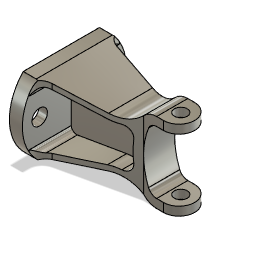
0.885.1264 - Pied de hauban - IGTE 21481_222676 (Autodesk Fusion 360 design; units mm, degrees)
Autodesk Fusion 360 part; units mm, degrees
sketch "Sketch1" plane through (0, 0, 0) normal (0, 0, 1) x (1, 0, 0)
  line L0 (0, 0) -> (0, 40)
  line L1 (0, 40) -> (15, 40)
  line L2 (0, 0) -> (0, -40)
  line L3 (0, -40) -> (15, -40)
  line L4 (15, 26.7964) -> (15, -26.7964)
  line L5 (15, 0) -> (85, 0) construction
  line L6 (85, 0) -> (85, 22) construction
  line L7 (85, 0) -> (85, -22) construction
  line L8 (79.9016, 28.874) -> (15, 40)
  line L9 (138, 0) -> (138, 68.5674) construction
  line L10 (113, 0) -> (113, 68.5674) construction
  line L11 (138, 46) -> (154, 46)
  line L12 (138, 36) -> (154, 36)
  line L13 (154, 46) -> (154, 36)
  line L14 (138, -36) -> (128.0077, -36)
  line L15 (138, -46) -> (154, -46)
  line L16 (138, -36) -> (154, -36)
  line L17 (154, -46) -> (154, -36)
  arc A0 (118.7231, 29.7143) -> (118.7231, -29.7143) centre (193, 0) ccw
  line L18 (138, 36) -> (128.0077, 36)
  arc A1 (128.0077, 36) -> (118.7231, 29.7143) centre (128.0077, 26) ccw
  arc A2 (118.7231, -29.7143) -> (128.0077, -36) centre (128.0077, -26) ccw
  arc A3 (128.0077, 46) -> (113.6334, 39.9061) centre (128.0077, 26) ccw
  line L19 (138, 46) -> (128.0077, 46)
  arc A4 (79.9016, 28.874) -> (113.6334, 39.9061) centre (86.3222, 66.3277) ccw
  line L20 (79.9016, -28.874) -> (15, -40)
  arc A5 (113.6334, -39.9061) -> (79.9016, -28.874) centre (86.3222, -66.3277) ccw
  arc A6 (113.6334, -39.9061) -> (128.0077, -46) centre (128.0077, -26) ccw
  line L21 (138, -46) -> (128.0077, -46)
  line L22 (78.8878, 22.9603) -> (22.0138, 32.7101)
  line L23 (78.8878, -22.9603) -> (22.0138, -32.7101)
  arc A7 (15, -26.7964) -> (22.0138, -32.7101) centre (21, -26.7964) ccw
  arc A8 (22.0138, 32.7101) -> (15, 26.7964) centre (21, 26.7964) ccw
  arc A9 (103.7464, 11.5668) -> (103.7464, -11.5668) centre (193, 0) ccw
  arc A10 (92.4391, -22.7549) -> (78.8878, -22.9603) centre (86.3222, -66.3277) ccw
  arc A11 (78.8878, 22.9603) -> (92.4391, 22.7549) centre (86.3222, 66.3277) ccw
  arc A12 (103.7464, 11.5668) -> (92.4391, 22.7549) centre (93.8293, 12.852) ccw
  arc A13 (92.4391, -22.7549) -> (103.7464, -11.5668) centre (93.8293, -12.852) ccw
  dimension "d1" = 40
  dimension "d2" = 15
  dimension "d3" = 40
  dimension "d4" = 15
  dimension "d5" = 70
  dimension "d6" = 22
  dimension "d7" = 22
  dimension "d10" = 138
  dimension "d11" = 36
  dimension "d13" = 25
  dimension "d14" = 16
  dimension "d15" = 16
  dimension "d16" = 160
  dimension "d17" = 10
  dimension "d18" = 10
  dimension "d20" = 38
  dimension "d23" = 6
  dimension "d24" = 6
  dimension "d28" = 10
  dimension "d29" = 10
  constraint coincident L0.start L2.start
  constraint perpendicular L3 L4
  constraint perpendicular L12 L13
  constraint symmetric L5 L12.start L14.start
  constraint symmetric L5 L11.start L15.start
  constraint symmetric L5 L11.end L15.end
  constraint symmetric L5 L12.end L16.end
  constraint coincident L10.start A0
  constraint tangent L18 A1
  constraint tangent A0 A1
  constraint tangent L14 A2
  constraint tangent A0 A2
  constraint concentric A1 A3
  constraint tangent L8 A4
  constraint tangent A3 A4
  constraint symmetric L1.end L5 L3.end
  constraint symmetric L5 A3.start A6.end
  constraint symmetric L5 A3 A6
  constraint symmetric L5 L8.start L20.start
  constraint symmetric L5 A3.end A5.start
  constraint symmetric L5 A4 A5
  constraint coincident L4 L5.start
  constraint parallel L8 L22
  constraint parallel L20 L23
  constraint tangent L23 A7
  constraint tangent L4 A7
  constraint tangent L4 A8
  constraint tangent L22 A8
  constraint concentric A4 A11
  constraint concentric A0 A9
  constraint concentric A5 A10
  constraint tangent A9 A12
  constraint tangent A11 A12
  constraint tangent A10 A13
  constraint tangent A9 A13
  measures "d1" distance of L0.start L0.end
  measures "d2" distance of L0.end L1.end
  measures "d3" distance of L0.start L2.end
  measures "d4" distance of L2.end L3.end
  measures "d5" distance of L5.start L5.end
  measures "d6" distance of L5.end L6.end
  measures "d10" distance of L0.start L9.start
  measures "d11" distance of L9.start L12.start
  measures "d14" distance of L11.start L11.end
  measures "d15" distance of L12.start L12.end
  measures "d16" diameter of A0
  measures "d17" radius of A1
  measures "d18" radius of A2
  measures "d20" radius of A4
  measures "d23" radius of A7
  measures "d24" radius of A8
  measures "d28" radius of A12
  measures "d29" radius of A13
extrude "Extrude1" add sketch "Sketch1" along normal mid plane 120
sketch "Sketch2" plane through (0, 0, 0) normal (0, 0, 1) x (1, 0, 0)
  line L0 (15, 26.7964) -> (15, -26.7964)
  line L1 (15, -26.7964) -> (15, 26.7964)
  arc A0 (22.0138, 32.7101) -> (15, 26.7964) centre (21, 26.7964) ccw
  arc A1 (22.0138, 32.7101) -> (15, 26.7964) centre (21, 26.7964) ccw
  line L2 (78.8878, 22.9603) -> (22.0138, 32.7101)
  line L3 (22.0138, 32.7101) -> (78.8878, 22.9603)
  arc A2 (78.8878, 22.9603) -> (92.4391, 22.7549) centre (86.3222, 66.3277) ccw
  arc A3 (78.8878, 22.9603) -> (92.4391, 22.7549) centre (86.3222, 66.3277) ccw
  arc A4 (103.7464, 11.5668) -> (92.4391, 22.7549) centre (93.8293, 12.852) ccw
  arc A5 (103.7464, 11.5668) -> (92.4391, 22.7549) centre (93.8293, 12.852) ccw
  arc A6 (103.7464, 11.5668) -> (103.7464, -11.5668) centre (193, 0) ccw
  arc A7 (103.7464, 11.5668) -> (103.7464, -11.5668) centre (193, 0) ccw
  arc A8 (92.4391, -22.7549) -> (103.7464, -11.5668) centre (93.8293, -12.852) ccw
  arc A9 (92.4391, -22.7549) -> (103.7464, -11.5668) centre (93.8293, -12.852) ccw
  arc A10 (92.4391, -22.7549) -> (78.8878, -22.9603) centre (86.3222, -66.3277) ccw
  arc A11 (92.4391, -22.7549) -> (78.8878, -22.9603) centre (86.3222, -66.3277) ccw
  line L4 (22.0138, -32.7101) -> (78.8878, -22.9603)
  line L5 (78.8878, -22.9603) -> (22.0138, -32.7101)
  arc A12 (15, -26.7964) -> (22.0138, -32.7101) centre (21, -26.7964) ccw
  arc A13 (15, -26.7964) -> (22.0138, -32.7101) centre (21, -26.7964) ccw
extrude "Extrude2" add sketch "Sketch2" along normal mid plane 7
sketch "Sketch3" plane through (0, 0, 0) normal (0, 1, 0) x (1, 0, 0)
  line L0 (128.0077, 60) -> (128.0077, -60) construction
  line L1 (128.0077, -60) -> (154, -60) construction
  line L2 (154, -60) -> (154, 60) construction
  line L3 (154, 60) -> (128.0077, 60) construction
  line L4 (113.6334, 60) -> (113.6334, -60) construction
  line L5 (113.6334, -60) -> (128.0077, -60) construction
  line L6 (128.0077, -60) -> (128.0077, 60) construction
  line L7 (128.0077, 60) -> (113.6334, 60) construction
  line L8 (79.9016, 60) -> (79.9016, -60) construction
  line L9 (113.6334, -60) -> (79.9016, -60) construction
  line L10 (113.6334, -60) -> (113.6334, 60) construction
  line L11 (79.9016, 60) -> (113.6334, 60) construction
  line L12 (15, 60) -> (15, -60) construction
  line L13 (15, -60) -> (79.9016, -60) construction
  line L14 (79.9016, -60) -> (79.9016, 60) construction
  line L15 (79.9016, 60) -> (15, 60) construction
  line L16 (0, 60) -> (0, -60)
  line L17 (0, -60) -> (15, -60)
  line L18 (15, -60) -> (15, 60) construction
  line L19 (15, 60) -> (0, 60)
  line L20 (154, 0) -> (0, 0) construction
  line L21 (136, 0) -> (136, 18) construction
  line L22 (136, 0) -> (136, -18) construction
  arc A0 (136, -18) -> (136, 18) centre (136, 0) ccw
  line L23 (136, 18) -> (113, 18)
  line L24 (136, -18) -> (113, -18)
  line L25 (154, 40) -> (0, 40) construction
  line L26 (154, -40) -> (0, -40) construction
  line L27 (113, 18) -> (26.7144, 37.3702)
  line L28 (113, -18) -> (26.7144, -37.3702)
  line L29 (15, 60) -> (15, 52.006)
  line L30 (15, -52.006) -> (15, -60)
  arc A1 (15, 52.006) -> (26.7144, 37.3702) centre (30, 52.006) ccw
  arc A2 (26.7144, -37.3702) -> (15, -52.006) centre (30, -52.006) ccw
  line L31 (15, 60) -> (154, 60)
  line L32 (154, 60) -> (154, 0)
  line L33 (154, 0) -> (154, -60)
  line L34 (154, -60) -> (15, -60)
  dimension "d34" = 36
  dimension "d35" = 23
  dimension "d36" = 23
  dimension "d37" = 40
  dimension "d38" = 40
  dimension "d39" = 15
  dimension "d40" = 15
  constraint midpoint L2 L20.start
  constraint coincident L20.end origin
  constraint coincident L20.start A0
  constraint coincident L21.start L22.start
  constraint perpendicular L20 L21
  constraint perpendicular L20 L22
  constraint coincident L12.start L15.end
  constraint perpendicular L25 L29
  constraint coincident L12.end L13.start
  constraint tangent L27 A1
  constraint tangent L29 A1
  constraint tangent L30 A2
  constraint tangent L28 A2
  constraint coincident L2.end L3.start
  constraint tangent A0 L32
  constraint coincident L1.end L2.start
  measures "d34" diameter of A0
  measures "d35" distance of L21.end L23.end
  measures "d36" distance of L22.end L24.end
  measures "d39" radius of A1
  measures "d40" radius of A2
extrude "Extrude3" cut sketch "Sketch3" along normal through all and the other way through all contours A0 L23 L27 L29 A1 L31 L32 | A0 L24 L28 L30 A2 L33 L34
sketch "Sketch4" plane through (0, 46, 0) normal (0, 1, 0) x (-1, 0, 0)
  line L0 (-128.0077, 18) -> (-136, 18)
  arc A0 (-136, 18) -> (-136, -18) centre (-136, 0) ccw
  line L1 (-136, -18) -> (-128.0077, -18)
  line L2 (-128.0077, -18) -> (-128.0077, 18)
  line L3 (-136, 18) -> (-128.0077, 18)
  line L4 (-128.0077, 18) -> (-128.0077, -18)
  line L5 (-128.0077, -18) -> (-136, -18)
  arc A1 (-136, 18) -> (-136, -18) centre (-136, 0) ccw
  line L6 (-136, -18) -> (-136, 18) construction
  line L7 (-138, -18) -> (-138, 18) construction
  circle A2 centre (-138, 0) radius 7.5
  dimension "d43" = 2
  dimension "d44" = 15
  constraint coincident A0.end L1.start
  constraint coincident L0.end A0.start
  constraint midpoint L7 A2.centre
  measures "d44" diameter of A2
extrude "Extrude4" cut sketch "Sketch4" against normal through all contours A2
sketch "Sketch5" plane through (0, 0, 0) normal (1, 0, 0) x (0, 0, -1)
  line L0 (60, -40) -> (-60, -40) construction
  line L1 (-60, -40) -> (-60, 40) construction
  line L2 (-60, 40) -> (60, 40) construction
  line L3 (60, 40) -> (60, -40) construction
  line L4 (60, 0) -> (-60, 0) construction
  circle A0 centre (-40, 0) radius 9
  line L5 (0, 40) -> (0, -40) construction
  circle A1 centre (40, 0) radius 9
  dimension "d49" = 18
  dimension "d50" = 40
  constraint midpoint L3 L4.start
  constraint midpoint L1 L4.end
  constraint coincident L4 A0.centre
  constraint midpoint L2 L5.start
  constraint midpoint L0 L5.end
  constraint symmetric A0 L5 A1
  measures "d49" diameter of A0
  measures "d50" horizontal distance of origin A0.centre
extrude "Extrude5" cut sketch "Sketch5" along normal through all
sketch "Sketch6" plane through (0, 0, 0) normal (1, 0, 0) x (0, 0, -1)
  circle A0 centre (40, 0) radius 9 construction
  circle A1 centre (-40, 0) radius 9 construction
  line L0 (60, -40) -> (-60, -40) construction
  line L1 (-60, -40) -> (-60, 40) construction
  line L2 (-60, 40) -> (60, 40) construction
  line L3 (60, 40) -> (60, -40) construction
  arc A2 (44, -40) -> (44, 40) centre (2, 0) ccw
  line L4 (44, 40) -> (60, 40)
  line L5 (44, -40) -> (60, -40)
  line L6 (60, 40) -> (60, -40)
  line L7 (0, 40) -> (0, -40) construction
  arc A3 (-44, 40) -> (-44, -40) centre (-2, 0) ccw
  line L8 (-44, 40) -> (-60, 40)
  line L9 (-60, 40) -> (-60, -40)
  line L10 (-44, -40) -> (-60, -40)
  constraint coincident L2 A2.end
  constraint coincident L0 A2.start
  constraint coincident L2.end L3.start
  constraint perpendicular L3 L4
  constraint coincident L0.start L3.end
  constraint perpendicular L3 L5
  constraint midpoint L2 L7.start
  constraint midpoint L0 L7.end
  constraint symmetric A2.end L7 A3.start
  constraint symmetric A2.start L7 A3.end
  constraint symmetric A2 L7 A3
  constraint symmetric L2.end L7 L1.end
  constraint symmetric L0.start L7 L0.end
extrude "Extrude6" cut sketch "Sketch6" along normal through all
sketch "Sketch7" plane through (0, 0, 0) normal (1, 0, 0) x (0, 0, -1)
  arc A0 (-44, 40) -> (-44, -40) centre (-2, 0) ccw construction
  line L0 (-44, 40) -> (44, 40) construction
  arc A1 (44, -40) -> (44, 40) centre (2, 0) ccw construction
  line L1 (44, -40) -> (-44, -40) construction
  circle A2 centre (40, 0) radius 9
  circle A3 centre (-40, 0) radius 9
  arc A4 (41.7995, -35) -> (41.7995, 35) centre (2, 0) ccw
  line L2 (-41.7995, 35) -> (41.7995, 35)
  arc A5 (-41.7995, 35) -> (-41.7995, -35) centre (-2, 0) ccw
  line L3 (41.7995, -35) -> (-41.7995, -35)
  dimension "d54" = 5
extrude "Extrude7" cut sketch "Sketch7" along normal blind 5
fillet "Fillet1" radius 5 4 edges at (5, 0, -55) (5, 35, 0) (5, -35, 0) (5, 0, 55)
